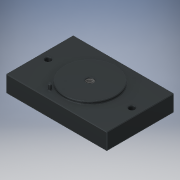
# Autodesk Inventor part: turningfixture
Saved by Autodesk Inventor 2017 (Build 210142000, 142)
## iProperties
Created: 2020-01-12
Part Number: turningfixture
Material: Iron, Cast
Document SubType Name: Modeling
Designer: Admin
Density: 7.15 g/cm^3
Appearance: Iron Gray
Author: Admin
Autodesk Inventor part; units mm, degrees
ref_plane "YZ Plane" through (0, 0, 0) normal (1, 0, 0) x (0, 1, 0)
ref_plane "XZ Plane" through (0, 0, 0) normal (0, 1, 0) x (-1, 0, 0)
ref_plane "XY Plane" through (0, 0, 0) normal (0, 0, 1) x (1, 0, 0)
sketch "Sketch1" plane through (0, 0, 0) normal (0, 1, 0) x (-1, 0, 0)
  line L0 (28.575, -19.05) -> (-28.575, -19.05)
  line L1 (-28.575, -19.05) -> (-28.575, 19.05)
  line L2 (-28.575, 19.05) -> (28.575, 19.05)
  line L3 (28.575, 19.05) -> (28.575, -19.05)
  point P0 (0, 0)
  dimension "d0" = 57.15
  dimension "d1" = 38.1
  dimension "d2" = 19.05
  dimension "d3" = 28.575
  constraints: 8 end point, 2 parallel, 1 horizontal, 1 perpendicular
  measures "d0" distance of L0.start L0.end
  measures "d1" distance of L2.end L0.start
  measures "d2" distance from line of point (0, 0) L0
  measures "d3" distance from line of point (0, 0) L3
extrude "Extrusion1" add sketch "Sketch1" along normal mid plane 11.1125
sketch "Sketch2" plane through (0, 5.5563, 0) normal (0, 1, 0) x (1, 0, 0)
  circle A0 centre (0, 0) radius 14.6844
  line L0 (28.575, 19.05) -> (-28.575, 19.05) projected
  line L1 (-28.575, -19.05) -> (28.575, -19.05) projected
  line L2 (-28.575, 19.05) -> (28.575, 19.05)
  line L3 (28.575, 19.05) -> (28.575, -19.05)
  line L4 (28.575, -19.05) -> (-28.575, -19.05)
  line L5 (-28.575, -19.05) -> (-28.575, 19.05)
  dimension "d6" = 29.3687
  constraints: 8 end point, 2 parallel, 1 centre point, 1 coincident, 1 horizontal, 1 perpendicular
  measures "d6" diameter of A0
extrude "Extrusion2" cut sketch "Sketch2" against normal blind 1.5875
sketch "Sketch3" plane through (0, 3.9688, 0) normal (0, 1, 0) x (1, 0, 0)
  line L0 (28.575, -19.05) -> (-28.575, -19.05) projected
  line L1 (-28.575, -19.05) -> (-28.575, 19.05) projected
  line L2 (28.575, 19.05) -> (28.575, -19.05) projected
  point P0 (0, 0)
  point P1 (-23.8125, 0)
  point P2 (23.8125, 0)
  dimension "d10" = 19.05
  dimension "d11" = 0
  dimension "d12" = 4.7625
  dimension "d13" = 4.7625
  measures "d10" distance from line of L0 point (-23.813, 0)
  measures "d11" vertical distance of point (-23.813, 0) point (23.813, 0)
  measures "d12" distance from line of L1 point (-23.813, 0)
  measures "d13" distance from line of L2 point (23.813, 0)
hole "Hole1" at (-23.8125, 3.9688, 0) at (23.8125, 3.9688, 0) direction (0, -1, 0) diameter 3.175 depth 25.4 tip angle 118
sketch "Sketch4" plane through (0, 5.5563, 0) normal (0, 1, 0) x (1, 0, 0)
  point P0 (0, 0)
  point P1 (0, 0)
  constraints: 1 coincident
hole "Hole2" at (0, 5.5563, 0) direction (0, -1, 0) diameter 4.0386 depth 25.4 tip angle 118
thread "Thread1" size "10-32 UNF" class "2B" standard "ANSI Unified Screw Threads" full length
sketch "Sketch6" plane through (0, 3.9688, 0) normal (0, 1, 0) x (1, 0, 0)
  circle A0 centre (-8.3312, -14.4272) radius 0.8255
  point P0 (0, 0)
  dimension "d33" = 1.651
  dimension "d34" = 14.4272
  dimension "d35" = 8.3312
  constraints: 1 centre point
  measures "d33" diameter of A0
  measures "d34" vertical distance of point (0, 0) A0.centre
  measures "d35" horizontal distance of A0.centre point (0, 0)
extrude "Extrusion3" add sketch "Sketch6" along normal blind 3.175
fillet "Fillet1" radius 0.3175 22 edges at (0, 3.9688, 19.05) (-28.575, -0.7938, 19.05) (0, -5.5563, 19.05) (28.575, -0.7937, 19.05) (0, 3.9688, -19.05) (-28.575, 3.9688, 0) (28.575, 3.9688, 0) (0, -5.5563, -19.05) (28.575, -5.5563, 0) (-28.575, -5.5563, 0) (28.575, -0.7937, -19.05) (-28.575, -0.7938, -19.05) (-23.8125, 3.9688, -1.5875) (23.8125, 3.9688, -1.5875) (0, 5.5563, -2.0193) (-14.6844, 3.9688, 0) (-14.6844, 5.5563, 0) (-9.1567, 7.1438, 14.4272) (0, -5.5563, -2.0193) (23.8125, -5.5563, -1.5875) (-23.8125, -5.5563, -1.5875) (-9.1567, 3.9688, 14.4272)
body "Solid1"
